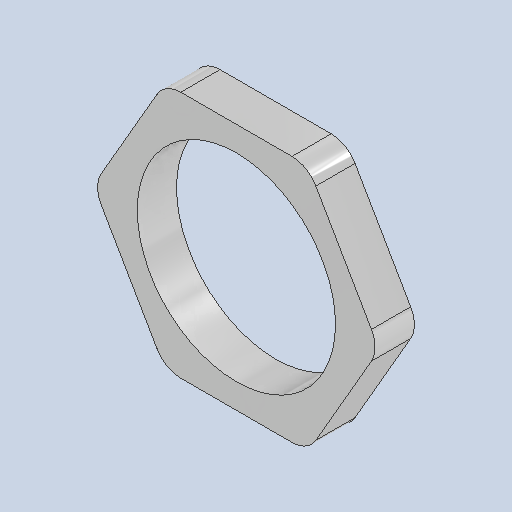
# Autodesk Inventor part: PG9x2.85mm_Nut
Saved by Autodesk Inventor 2024.2 (Build 282272000, 272)
## iProperties
Created: 2020-07-14
Part Number: PG9x2.85mm_Nut
Material: Generic
Document SubType Name: Modeling
Designer: CASE-SMALL2
Density: 1 g/cm^3
Appearance: Default
Author: CASE-SMALL2
Autodesk Inventor part; units mm, degrees
ref_plane "YZ Plane" through (0, 0, 0) normal (1, 0, 0) x (0, 1, 0)
ref_plane "XZ Plane" through (0, 0, 0) normal (0, 1, 0) x (-1, 0, 0)
ref_plane "XY Plane" through (0, 0, 0) normal (0, 0, 1) x (1, 0, 0)
sketch "Sketch1" plane through (0, 0, 0) normal (0, 0, 1) x (1, 0, 0)
  line L0 (10.3923, 0) -> (5.1962, -9)
  line L1 (5.1962, -9) -> (-5.1962, -9)
  line L2 (-5.1962, -9) -> (-10.3923, 0)
  line L3 (-10.3923, 0) -> (-5.1962, 9)
  line L4 (-5.1962, 9) -> (5.1962, 9)
  line L5 (5.1962, 9) -> (10.3923, 0)
  circle A0 centre (0, 0) radius 7.2
  dimension "d0" = 18
  dimension "d1" = 14.4
  constraints: 12 end point, 2 coincident, 1 centre point, 13 other
  measures "d0" distance between parallel lines of L4 L1
  measures "d1" diameter of A0
extrude "Extrusion1" add sketch "Sketch1" along normal blind 2.85
fillet "Fillet1" radius 2 6 edges at (-5.1962, 9, 1.425) (5.1962, 9, 1.425) (10.3923, 0, 1.425) (-5.1962, -9, 1.425) (-10.3923, 0, 1.425) (5.1962, -9, 1.425)
body "Solid1"
